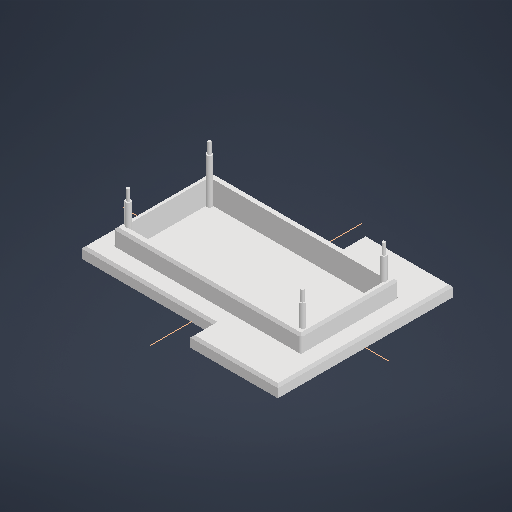
# Autodesk Inventor part: Buggy_Body_Wheel_Wells
Saved by Autodesk Inventor 2026.2 (Build 302298010, 298A)
## iProperties
Created: 2026-02-09
Part Number: Buggy_Body_Wheel_Wells
Material: Generic
Document SubType Name: Modeling
Designer: dm2166
Density: 1 g/cm^3
Appearance: Default
Author: dm2166
Autodesk Inventor part; units mm, degrees
ref_plane "YZ Plane" through (0, 0, 0) normal (1, 0, 0) x (0, 1, 0)
ref_plane "XZ Plane" through (0, 0, 0) normal (0, 1, 0) x (-1, 0, 0)
ref_plane "XY Plane" through (0, 0, 0) normal (0, 0, 1) x (1, 0, 0)
sketch "Sketch1" plane through (0, 0, 0) normal (0, 1, 0) x (-1, 0, 0)
  line L0 (-85.5, -44.5) -> (85.5, -44.5)
  line L1 (85.5, -44.5) -> (85.5, 44.5)
  line L2 (85.5, 44.5) -> (-85.5, 44.5)
  line L3 (-85.5, 44.5) -> (-85.5, -44.5)
  line L4 (-85.5, -44.5) -> (85.5, 44.5) construction
  line L5 (85.5, -44.5) -> (-85.5, 44.5) construction
  line L6 (-81, -38.5) -> (81, -38.5)
  line L7 (81, -38.5) -> (81, 38.5)
  line L8 (81, 38.5) -> (-81, 38.5)
  line L9 (-81, 38.5) -> (-81, -38.5)
  line L10 (-81, -38.5) -> (81, 38.5) construction
  line L11 (81, -38.5) -> (-81, 38.5) construction
  line L12 (81, 38.5) -> (79.55, 38.5)
  line L13 (81, 37.05) -> (81, 38.5)
  circle A0 centre (79.55, 37.05) radius 1.45
  circle A1 centre (79.55, -37.05) radius 1.45
  circle A2 centre (-79.55, -37.05) radius 1.45
  circle A3 centre (-79.55, 37.05) radius 1.45
  line L14 (81, 38.5) -> (78.1, 38.5)
  line L15 (78.1, 38.5) -> (78.1, 35.6)
  line L16 (78.1, 35.6) -> (81, 35.6)
  line L17 (81, 35.6) -> (81, 38.5)
  line L18 (81, 38.5) -> (78.1, 35.6) construction
  line L19 (78.1, 38.5) -> (81, 35.6) construction
  line L20 (81, -35.6) -> (78.1, -35.6)
  line L21 (78.1, -35.6) -> (78.1, -38.5)
  line L22 (78.1, -38.5) -> (81, -38.5)
  line L23 (81, -38.5) -> (81, -35.6)
  line L24 (81, -35.6) -> (78.1, -38.5) construction
  line L25 (78.1, -35.6) -> (81, -38.5) construction
  line L26 (-81, -38.5) -> (-78.1, -38.5)
  line L27 (-78.1, -35.6) -> (-81, -38.5) construction
  line L28 (-81, -35.6) -> (-78.1, -38.5) construction
  line L29 (-78.1, 38.5) -> (-81, 38.5)
  line L30 (-81, 38.5) -> (-81, 35.6)
  line L31 (-78.1, 38.5) -> (-81, 35.6) construction
  line L32 (-81, 38.5) -> (-78.1, 35.6) construction
  circle A4 centre (-79.55, 37.05) radius 2.5
  line L33 (-95.5566, 0) -> (75.4434, 0)
  line L34 (0, 31.9167) -> (0, -57.0833)
  circle A5 centre (-79.55, -37.05) radius 2.5
  circle A6 centre (79.55, 37.05) radius 2.5
  circle A7 centre (79.55, -37.05) radius 2.5
  line L35 (140, 0) -> (-140, 0) projected
  line L36 (0, -112) -> (0, 112) projected
  line L37 (-100, 59.2475) -> (100, 59.2475)
  line L38 (100, 59.2475) -> (100, -59.2475)
  line L39 (100, -59.2475) -> (-100, -59.2475)
  line L40 (-100, -59.2475) -> (-100, 59.2475)
  line L41 (-100, 59.2475) -> (100, -59.2475) construction
  line L42 (100, 59.2475) -> (-100, -59.2475) construction
  line L43 (-100, 80) -> (-20, 80)
  line L44 (-20, 80) -> (-20, -80)
  line L45 (-20, -80) -> (-100, -80)
  line L46 (-100, -80) -> (-100, 80)
  line L47 (-100, 80) -> (-20, -80) construction
  line L48 (-20, 80) -> (-100, -80) construction
  point P0 (0, 0)
  point P1 (-79.55, 38.5)
  point P2 (-81, 37.05)
  point P3 (-81, -37.05)
  point P4 (-79.55, -38.5)
  point P5 (79.55, -38.5)
  point P6 (81, -37.05)
  point P7 (-60, 0)
  point P8 (-20, 59.2475)
  point P9 (-20, -59.2475)
  dimension "d0" = 171
  dimension "d1" = 89
  dimension "d2" = 162
  dimension "d3" = 77
  dimension "d7" = 2.9
  dimension "d8" = 2.9
  dimension "d9" = 2.9
  dimension "d10" = 2.9
  dimension "d53" = 5
  dimension "d56" = 200
  dimension "d57" = 80
  dimension "d58" = 160
  constraints: 94 end point, 16 midpoint, 14 parallel, 8 centre point, 8 horizontal, 8 perpendicular, 8 tangent, 6 point on line, 3 collinear, 3 symmetric about line, 1 coincident, 1 vertical, 3 other
  measures "d0" distance of L2.end L1.end
  measures "d1" distance of L1.end L0.end
  measures "d2" distance of L8.end L7.end
  measures "d3" distance of L7.end L6.end
  measures "d7" diameter of A0
  measures "d8" diameter of A1
  measures "d9" diameter of A2
  measures "d10" diameter of A3
  measures "d53" diameter of A4
  measures "d56" distance of L38.end L39.end
  measures "d57" distance of L44.end L45.end
  measures "d58" distance of L43.end L44.end
extrude "Extrusion1" add sketch "Sketch1" along normal blind 55 contours A2 | A3 | A1 | A0
extrude "Extrusion2" add sketch "Sketch1" along normal blind 4 contours L44 L33 L34 L6 | L6 A5 L9 L33 L44 | L9 A4 L8 L44 L33 | L34 L33 L35 L7 A7 L6 | L6 A2 L9 A5 | L44 L8 L36 L34 L33 | L9 A3 L8 A4 | A7 L7 L20 L21 L6 | L34 L36 L8 A6 L7 L35 L33 | L21 A1 L6 | A6 L8 L15 L16 L7 | L21 L20 A1 | L7 A1 L20 | L16 A0 L7 | L8 A0 L15 | L16 L15 A0
extrude "Extrusion3" add sketch "Sketch1" along normal blind 25 contours L3 L33 L9 A5 L6 L44 L0 | L44 L6 L34 L0 | L3 L2 L44 L8 A4 L9 L33 | L34 L6 A7 L7 L35 L1 L0 | A5 L9 L6 | L2 L36 L8 L44 | A4 L8 L9 | L35 L7 A6 L8 L36 L2 L1 | L6 L7 A7 | L7 L8 A6
chamfer "Chamfer1" distance 2 angle 45 4 edges at (0, 25, 44.5) (85.5, 25, 0) (0, 25, -44.5) (-85.5, 25, 0)
fillet "Fillet6" radius 2 1 edges at (85.5, 11.5, 44.5)
fillet "Fillet7" radius 2 1 edges at (85.5, 11.5, -44.5)
fillet "Fillet8" radius 2 1 edges at (-85.5, 11.5, 44.5)
fillet "Fillet9" radius 2 1 edges at (-85.5, 11.5, -44.5)
extrude "Extrusion11" add sketch "Sketch1" along normal blind 45 contours A5 L9 L6 | L6 A2 L9 A5 | A4 L8 L9 | L9 A3 L8 A4 | A7 L7 L20 L21 L6 | L6 L7 A7 | A2 L6 L9 | A2 | L21 A1 L6 | L9 L8 A3 | A3 | A6 L8 L15 L16 L7 | L7 L8 A6 | A1 L7 L6 | A1 | L21 L20 A1 | L7 A1 L20 | L16 A0 L7 | L8 A0 L15 | A0 L8 L7 | A0 | L16 L15 A0
extrude "Extrusion12" add sketch "Sketch1" along normal blind 10 contours L0 L44 L39 L40 L35 L33 L3 | L0 L34 L36 L39 L44 | L33 L35 L40 L37 L44 L2 L3 | L0 L1 L35 L38 L39 L36 L34 | L44 L45 L46 L39 | L44 L37 L36 L2 | L1 L2 L36 L37 L38 L35 | L37 L46 L43 L44
chamfer "Chamfer2" distance 2 angle 45 8 edges at (100, 10, 0) (60, 10, 80) (20, 10, 69.6238) (60, 10, -80) (20, 10, -69.6238) (-40, 10, -59.2475) (-40, 10, 59.2475) (-100, 10, 0)
sketch "Sketch4" plane through (0, 0, 0) normal (0, -1, 0) x (1, 0, 0)
  circle A0 centre (-11.2675, 0) radius 2 projected
  circle A1 centre (-71.2675, 0) radius 2 projected
  circle A2 centre (-41.2675, 30) radius 2 projected
  circle A3 centre (-11.2675, 0) radius 1.9
  circle A4 centre (-71.2675, 0) radius 1.9
  circle A5 centre (-41.2675, 30) radius 1.9
  point P0 (0, 0)
  dimension "d64" = 3.8
  constraints: 3 centre point, 3 coincident, 2 equal radius
  measures "d64" diameter of A5
extrude "Extrusion13" add sketch "Sketch4" along normal blind 10 contours A3 | A4 | A5
body "Solid1"
